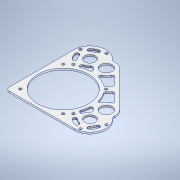
# Autodesk Inventor part: TopPlate
Saved by Autodesk Inventor 2020 (Build 240168000, 168)
## iProperties
Created: 2019-06-07
Part Number: TopPlate
Material: Aluminum 6061
Document SubType Name: Modeling
Designer: Connor
Density: 2.7 g/cm^3
Appearance: Aluminum - Flat
Author: Connor
Autodesk Inventor part; units mm, degrees
ref_plane "YZ Plane" through (0, 0, 0) normal (1, 0, 0) x (0, 1, 0)
ref_plane "XZ Plane" through (0, 0, 0) normal (0, 1, 0) x (-1, 0, 0)
ref_plane "XY Plane" through (0, 0, 0) normal (0, 0, 1) x (1, 0, 0)
sketch "Sketch1" plane through (0, 0, 0) normal (0, 1, 0) x (-1, 0, 0)
  circle A0 centre (0, 0) radius 48.26
  circle A1 centre (0, 0) radius 57.15 construction
  circle A2 centre (40.4112, -40.4112) radius 2.4892
  circle A3 centre (-40.4112, -40.4112) radius 2.4892
  circle A4 centre (-40.4112, 40.4112) radius 2.4892
  circle A5 centre (40.4112, 40.4112) radius 2.4892
  line L0 (40.4112, -40.4112) -> (40.4112, 40.4112) construction
  line L1 (40.4112, 40.4112) -> (-40.4112, 40.4112) construction
  line L2 (53.975, 53.975) -> (-111.125, 53.975)
  line L3 (-111.125, 53.975) -> (-111.125, -111.125)
  line L4 (-111.125, -111.125) -> (53.975, -111.125)
  line L5 (53.975, -111.125) -> (53.975, 53.975)
  circle A6 centre (0, 0) radius 53.975 construction
  dimension "d0" = 96.52
  dimension "d1" = 114.3
  dimension "d2" = 4.9784
  dimension "d3" = 107.95
  dimension "d8" = 165.1
  constraints: 12 end point, 7 centre point, 4 perpendicular, 4 point on circle, 3 coincident, 3 equal radius, 2 horizontal alignment, 2 parallel, 2 tangent, 1 horizontal, 1 vertical, 1 vertical alignment
  measures "d0" diameter of A0
  measures "d1" diameter of A1
  measures "d2" diameter of A2
  measures "d3" diameter of A6
  measures "d8" distance of L4.end L2.start
extrude "Extrusion1" add sketch "Sketch1" along normal blind 3.175
sketch "Sketch2" plane through (0, 3.175, 0) normal (0, 1, 0) x (1, 0, 0)
  circle A0 centre (0, 0) radius 75.05 construction
  circle A1 centre (6.5038, 74.7677) radius 22.86 construction
  circle A2 centre (-23.975, 74.4972) radius 7.62 construction
  circle A3 centre (-23.975, 74.4972) radius 30 construction
  line L0 (-53.975, 111.125) -> (-53.975, -53.975) construction
  circle A4 centre (-40.4112, 40.4112) radius 2.4892 construction
  circle A5 centre (-23.975, 74.4972) radius 10
  circle A6 centre (6.5038, 74.7677) radius 11.1125
  circle A7 centre (-23.975, 74.4972) radius 25.4 construction
  line L1 (-53.975, -53.975) -> (111.125, -53.975) construction
  line L2 (111.125, -53.975) -> (111.125, 111.125) construction
  line L3 (-53.975, -53.975) -> (111.125, 111.125) construction
  circle A8 centre (74.4972, -23.975) radius 10
  circle A9 centre (74.7677, 6.5038) radius 11.1125
  line L4 (-48.5095, 81.0712) -> (-17.401, 99.0317) construction
  line L5 (-17.401, 99.0317) -> (0.5595, 67.9232) construction
  line L6 (0.5595, 67.9232) -> (-30.549, 49.9626) construction
  line L7 (-30.549, 49.9626) -> (-48.5095, 81.0712) construction
  circle A10 centre (-48.5095, 81.0712) radius 2.4892
  circle A11 centre (40.4112, -40.4112) radius 2.4892 construction
  circle A12 centre (40.4112, -40.4112) radius 2.4892
  circle A13 centre (81.0712, -48.5095) radius 2.4892
  circle A14 centre (-17.401, 99.0317) radius 2.4892
  circle A15 centre (0.5595, 67.9232) radius 2.4892
  circle A16 centre (99.0317, -17.401) radius 2.4892
  circle A17 centre (67.9232, 0.5595) radius 2.4892
  line L8 (111.125, 111.125) -> (-53.975, 111.125) projected
  circle A18 centre (0, 0) radius 48.26 projected
  circle A19 centre (-30.549, 49.9626) radius 2.4892
  circle A20 centre (49.9626, -30.549) radius 2.4892
  point P0 (-6.6266, 81.4577)
  point P1 (-8.533, 76.8596)
  point P2 (81.4577, -6.6266)
  point P3 (76.8596, -8.533)
  dimension "d9" = 150.1
  dimension "d10" = 45.72
  dimension "d11" = 15.24
  dimension "d13" = 60
  dimension "d16" = 20
  dimension "d17" = 50.8
  dimension "d18" = 22.225
  dimension "d114" = 30
  constraints: 18 centre point, 10 coincident, 10 end point, 7 symmetric about line, 4 equal radius, 3 point on circle, 3 tangent, 2 parallel, 2 perpendicular, 10 other
  measures "d10" diameter of A1
  measures "d11" diameter of A2
  measures "d13" diameter of A3
  measures "d16" diameter of A5
  measures "d17" diameter of A7
  measures "d18" diameter of A6
  measures "d114" angle of L0 L7
extrude "Extrusion2" cut sketch "Sketch2" against normal blind 6.35 contours A5 | A6 A15 | A15 A6 | A8 | A9 A17 | A17 A9 | A10 | A12 | A13 | A14 | A16 | A19 | A20 picked at (9.8961, 78.6539) picked at (0.154, 67.5729) picked at (79.0892, 9.3447) picked at (67.5155, 0.2253)
sketch "Sketch5" plane through (0, 3.175, 0) normal (0, 1, 0) x (1, 0, 0)
  circle A0 centre (-23.975, 74.4972) radius 10 projected
  line L0 (-53.975, 111.125) -> (-53.975, -53.975) projected
  arc A1 (-2.7618, 95.7104) -> (-53.975, 74.4972) centre (-23.975, 74.4972) ccw
  circle A2 centre (74.4972, -23.975) radius 10 projected
  line L1 (-53.975, -53.975) -> (111.125, -53.975) projected
  arc A3 (74.4972, -53.975) -> (95.7104, -2.7618) centre (74.4972, -23.975) ccw
  circle A4 centre (6.5038, 74.7677) radius 11.1125 projected
  circle A5 centre (6.5038, 74.7677) radius 17.4625
  circle A6 centre (74.7677, 6.5038) radius 11.1125 projected
  circle A7 centre (74.7677, 6.5038) radius 17.4625
  line L2 (18.8517, 87.1155) -> (87.1155, 18.8517)
  line L3 (111.125, 111.125) -> (-53.975, 111.125) projected
  line L4 (111.125, -53.975) -> (111.125, 111.125) projected
  line L5 (-2.7618, 95.7104) -> (95.7104, -2.7618)
  point P0 (0, 0)
  point P1 (13.193, 90.8982)
  point P2 (90.8982, 13.193)
  point P3 (1.4621, 91.4865)
  point P4 (91.4865, 1.4621)
  point P5 (23.2226, 69.7259)
  point P6 (69.7259, 23.2226)
  dimension "d70" = 34.925
  constraints: 8 point on circle, 6 tangent, 4 centre point, 4 coincident, 4 end point, 2 point on line, 1 equal radius
  measures "d70" diameter of A5
extrude "Extrusion5" cut sketch "Sketch5" against normal blind 6.35 contours L3 L4 L1 A3 L5 A7 L2 A5 A1 L0
fillet "Fillet3" radius 6.35 3 edges at (-53.975, 1.5875, 53.975) (91.4865, 1.5875, -1.4621) (1.4621, 1.5875, -91.4865)
sketch "Sketch6" plane through (0, 3.175, 0) normal (0, 1, 0) x (1, 0, 0)
  circle A0 centre (6.5038, 74.7677) radius 11.1125 projected
  arc A1 (13.5073, 58.7711) -> (22.651, 68.1188) centre (6.5038, 74.7677) ccw
  circle A2 centre (74.7677, 6.5038) radius 11.1125 projected
  circle A3 centre (40.4112, 40.4112) radius 2.4892 construction
  line L0 (0, 0) -> (40.4112, 40.4112) construction
  line L1 (35.8111, 44.7914) -> (41.7583, 50.7385)
  line L2 (27.8319, 69.155) -> (41.7583, 55.2286)
  arc A4 (31.7218, 44.452) -> (13.9686, 52.7933) centre (0, 0) ccw
  line L3 (87.1155, 18.8517) -> (18.8517, 87.1155) projected
  circle A5 centre (0, 0) radius 48.26 projected
  arc A6 (13.5073, 58.7711) -> (13.9686, 52.7933) centre (14.7807, 55.8627) ccw
  arc A7 (31.7218, 44.452) -> (35.8111, 44.7914) centre (33.5661, 47.0364) ccw
  arc A8 (41.7583, 50.7385) -> (41.7583, 55.2286) centre (39.5132, 52.9836) ccw
  arc A9 (27.8319, 69.155) -> (22.651, 68.1188) centre (25.5868, 66.9099) ccw
  circle A10 centre (-23.975, 74.4972) radius 10 projected
  arc A11 (-20.5149, 58.5175) -> (-11.7303, 63.6625) centre (-23.975, 74.4972) ccw
  arc A12 (-6.9131, 63.5907) -> (-3.1566, 60.2207) centre (6.5038, 74.7677) ccw
  arc A13 (-4.6431, 54.4123) -> (-18.3313, 51.4414) centre (0, 0) ccw
  circle A14 centre (-30.549, 49.9626) radius 2.4892 projected
  arc A15 (-22.3442, 53.251) -> (-22.6723, 53.9737) centre (-30.549, 49.9626) ccw
  arc A16 (-6.9131, 63.5907) -> (-11.7303, 63.6625) centre (-9.3526, 61.5585) ccw
  arc A17 (-20.5149, 58.5175) -> (-22.6723, 53.9737) centre (-19.843, 55.4144) ccw
  arc A18 (-22.3442, 53.251) -> (-18.3313, 51.4414) centre (-19.3971, 54.4321) ccw
  arc A19 (-4.6431, 54.4123) -> (-3.1566, 60.2207) centre (-4.9131, 57.5758) ccw
  line L4 (-53.975, 74.4972) -> (-53.975, -47.625) projected
  circle A20 centre (-48.5095, 81.0712) radius 2.4892 projected
  circle A21 centre (-40.4112, 40.4112) radius 2.4892 projected
  circle A22 centre (-17.401, 99.0317) radius 2.4892 projected
  arc A23 (-2.7618, 95.7104) -> (-53.975, 74.4972) centre (-23.975, 74.4972) ccw projected
  arc A24 (68.1188, 22.651) -> (58.7711, 13.5073) centre (74.7677, 6.5038) ccw
  line L5 (44.7914, 35.8111) -> (50.7385, 41.7583)
  line L6 (69.155, 27.8319) -> (55.2286, 41.7583)
  arc A25 (52.7933, 13.9686) -> (44.452, 31.7218) centre (0, 0) ccw
  arc A26 (52.7933, 13.9686) -> (58.7711, 13.5073) centre (55.8627, 14.7807) ccw
  arc A27 (44.7914, 35.8111) -> (44.452, 31.7218) centre (47.0364, 33.5661) ccw
  arc A28 (55.2286, 41.7583) -> (50.7385, 41.7583) centre (52.9836, 39.5132) ccw
  arc A29 (68.1188, 22.651) -> (69.155, 27.8319) centre (66.9099, 25.5868) ccw
  arc A30 (63.6625, -11.7303) -> (58.5175, -20.5149) centre (74.4972, -23.975) ccw
  arc A31 (60.2207, -3.1566) -> (63.5907, -6.9131) centre (74.7677, 6.5038) ccw
  arc A32 (51.4414, -18.3313) -> (54.4123, -4.6431) centre (0, 0) ccw
  arc A33 (53.9737, -22.6723) -> (53.251, -22.3442) centre (49.9626, -30.549) ccw
  arc A34 (63.6625, -11.7303) -> (63.5907, -6.9131) centre (61.5585, -9.3526) ccw
  arc A35 (53.9737, -22.6723) -> (58.5175, -20.5149) centre (55.4144, -19.843) ccw
  arc A36 (51.4414, -18.3313) -> (53.251, -22.3442) centre (54.4321, -19.3971) ccw
  arc A37 (60.2207, -3.1566) -> (54.4123, -4.6431) centre (57.5758, -4.9131) ccw
  line L7 (-23.975, 74.4972) -> (-48.5095, 81.0712) construction
  line L8 (-23.975, 74.4972) -> (-17.401, 99.0317) construction
  line L9 (-39.8385, 85.3218) -> (-38.7948, 85.0421)
  line L10 (-25.4176, 93.6477) -> (-25.6973, 92.604)
  arc A38 (-29.1837, 97.5664) -> (-41.3492, 90.5427) centre (-23.975, 74.4972) ccw
  arc A39 (-27.9853, 90.3477) -> (-35.6968, 85.8955) centre (-23.975, 74.4972) ccw
  arc A40 (-41.3492, 90.5427) -> (-39.8385, 85.3218) centre (-39.0167, 88.3886) ccw
  arc A41 (-38.7948, 85.0421) -> (-35.6968, 85.8955) centre (-37.973, 88.1089) ccw
  arc A42 (-25.4176, 93.6477) -> (-29.1837, 97.5664) centre (-28.4845, 94.4694) ccw
  arc A43 (-27.9853, 90.3477) -> (-25.6973, 92.604) centre (-28.7641, 93.4257) ccw
  line L11 (85.3218, -39.8385) -> (85.0421, -38.7948)
  line L12 (93.6477, -25.4176) -> (92.604, -25.6973)
  arc A44 (90.5427, -41.3492) -> (97.5664, -29.1837) centre (74.4972, -23.975) ccw
  arc A45 (85.8955, -35.6968) -> (90.3477, -27.9853) centre (74.4972, -23.975) ccw
  arc A46 (85.3218, -39.8385) -> (90.5427, -41.3492) centre (88.3886, -39.0167) ccw
  arc A47 (85.8955, -35.6968) -> (85.0421, -38.7948) centre (88.1089, -37.973) ccw
  arc A48 (97.5664, -29.1837) -> (93.6477, -25.4176) centre (94.4694, -28.4845) ccw
  arc A49 (92.604, -25.6973) -> (90.3477, -27.9853) centre (93.4257, -28.7641) ccw
  line L13 (-23.975, 74.4972) -> (-30.549, 49.9626) construction
  line L14 (-43.1255, 73.0545) -> (-42.0818, 72.7749)
  line L15 (-34.52, 59.6774) -> (-34.7996, 58.6337)
  arc A50 (-47.0443, 69.2884) -> (-40.0205, 57.1229) centre (-23.975, 74.4972) ccw
  arc A51 (-39.8255, 70.4868) -> (-35.3733, 62.7754) centre (-23.975, 74.4972) ccw
  arc A52 (-43.1255, 73.0545) -> (-47.0443, 69.2884) centre (-43.9472, 69.9877) ccw
  arc A53 (-39.8255, 70.4868) -> (-42.0818, 72.7749) centre (-42.9035, 69.708) ccw
  arc A54 (-34.52, 59.6774) -> (-35.3733, 62.7754) centre (-37.5868, 60.4991) ccw
  arc A55 (-40.0205, 57.1229) -> (-34.7996, 58.6337) centre (-37.8664, 59.4554) ccw
  line L16 (73.0545, -43.1255) -> (72.7749, -42.0818)
  line L17 (59.6774, -34.52) -> (58.6337, -34.7996)
  arc A56 (57.1229, -40.0205) -> (69.2884, -47.0443) centre (74.4972, -23.975) ccw
  arc A57 (62.7754, -35.3733) -> (70.4868, -39.8255) centre (74.4972, -23.975) ccw
  arc A58 (69.2884, -47.0443) -> (73.0545, -43.1255) centre (69.9877, -43.9472) ccw
  arc A59 (72.7749, -42.0818) -> (70.4868, -39.8255) centre (69.708, -42.9035) ccw
  arc A60 (62.7754, -35.3733) -> (59.6774, -34.52) centre (60.4991, -37.5868) ccw
  arc A61 (58.6337, -34.7996) -> (57.1229, -40.0205) centre (59.4554, -37.8664) ccw
  point P0 (-47.6238, 74.2598)
  point P1 (-40.1716, 72.263)
  point P2 (-36.0049, 54.1354)
  point P3 (-34.0081, 61.5875)
  dimension "d72" = 6.35
  dimension "d73" = 6.35
  dimension "d74" = 6.35
  dimension "d76" = 3.175
  dimension "d77" = 6.35
  dimension "d78" = 6.35
  dimension "d79" = 6.35
  dimension "d82" = 6.35
  dimension "d83" = 6.35
  dimension "d102" = 6.35
  dimension "d103" = 6.35
  dimension "d104" = 6.35
  dimension "d105" = 6.35
  dimension "d110" = 6.35
  dimension "d111" = 6.35
  dimension "d112" = 6.35
  constraints: 108 point on circle, 56 symmetric about line, 52 centre point, 32 end point, 32 tangent, 16 equal radius, 12 coincident, 6 parallel, 4 point on line, 26 other
  measures "d72" radial gap between concentric circles of A0 A1
  measures "d73" distance between parallel lines of L3 L2
  measures "d74" radial gap between concentric circles of A5 A4
  measures "d76" radius of A9
  measures "d77" distance between parallel lines of L1 L0
  measures "d78" radial gap between concentric circles of A0 A12
  measures "d79" radial gap between concentric circles of A10 A11
  measures "d82" radial gap between concentric circles of A14 A15
  measures "d83" radial gap between concentric circles of A5 A13
  measures "d102" distance between parallel lines of L7 L9
  measures "d103" distance between parallel lines of L8 L10
  measures "d104" radial gap between concentric circles of A23 A38
  measures "d105" radial gap between concentric circles of A10 A39
  measures "d110" distance between parallel lines of L14 L7
  measures "d111" distance between parallel lines of L13 L15
  measures "d112" radial gap between concentric circles of A10 A51
extrude "Extrusion6" cut sketch "Sketch6" against normal through all contours A1 A9 L2 A8 L1 A7 A4 A6 | A11 A16 A12 A19 A13 A18 A15 A17 | A24 A26 A25 A27 L5 A28 L6 A29 | A30 A35 A33 A36 A32 A37 A31 A34 | A40 A38 A42 L10 A43 A39 A41 L9 | L11 A47 A45 A49 L12 A48 A44 A46 | L14 A53 A51 A54 L15 A55 A50 A52 | A58 A56 A61 L17 A60 A57 A59 L16
body "Solid1"
